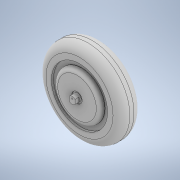
# Autodesk Inventor part: motor at24v
Saved by Autodesk Inventor 2022.2 (Build 262287010, 287A)
## iProperties
Created: 2022-03-16
Part Number: motor at24v
Material: Generic
Document SubType Name: Modeling
Designer: Finn Oriwohl
Density: 1 g/cm^3
Appearance: Default
Author: Finn Oriwohl
Autodesk Inventor part; units mm, degrees
ref_plane "YZ Plane" through (0, 0, 0) normal (1, 0, 0) x (0, 1, 0)
ref_plane "XZ Plane" through (0, 0, 0) normal (0, 1, 0) x (-1, 0, 0)
ref_plane "XY Plane" through (0, 0, 0) normal (0, 0, 1) x (1, 0, 0)
sketch "Sketch1" plane through (0, 0, 0) normal (0, 0, 1) x (1, 0, 0)
  circle A0 centre (0, 0) radius 100
  circle A1 centre (0, 0) radius 56
  circle A2 centre (0, 0) radius 67
  circle A3 centre (0, 0) radius 7.5
  dimension "d0" = 200
  dimension "d1" = 112
  dimension "d2" = 11
  dimension "d3" = 15
  constraints: 4 centre point, 3 coincident
  measures "d0" diameter of A0
  measures "d1" diameter of A1
  measures "d2" radial gap between concentric circles of A1 A2
  measures "d3" diameter of A3
extrude "Extrusion1" [suppressed]
extrude "Extrusion2" [suppressed]
extrude "Extrusion3" [suppressed]
extrude "Extrusion4" [suppressed]
sketch "Sketch2" plane through (0, 0, 0) normal (1, 0, 0) x (0, 1, 0)
  line L0 (0, 42.5) -> (0, -42.5)
  line L1 (0, 42.5) -> (8.5, 42.5)
  line L2 (8.5, 42.5) -> (8.5, -42.5)
  line L3 (8.5, -42.5) -> (0, -42.5)
  line L4 (56, 31) -> (56, -31)
  line L5 (0, 0) -> (100, 0) construction
  line L6 (56, 31) -> (12.3593, 31)
  line L7 (56, -31) -> (12.3593, -31)
  line L8 (67, 20) -> (67, -20)
  line L9 (100, 25) -> (100, -25)
  line L10 (56, 20) -> (67, 20)
  line L11 (67, -20) -> (56, -20)
  line L12 (100, 25) -> (67, 25)
  line L13 (67, 25) -> (67, 20)
  line L14 (67, -20) -> (67, -25)
  line L15 (67, -25) -> (100, -25)
  line L16 (12.3593, 31) -> (12.3593, 29.5)
  line L17 (12.3593, 29.5) -> (8.5, 29.5)
  line L18 (12.3593, -31) -> (12.3593, -29.5)
  line L19 (12.3593, -29.5) -> (8.5, -29.5)
  point P0 (56, 0)
  point P1 (8.5, 32.5)
  point P2 (8.5, -32.5)
  point P3 (67, 0)
  point P4 (4.25, 42.5)
  dimension "d12" = 85
  dimension "d13" = 8.5
  dimension "d15" = 100
  dimension "d16" = 56
  dimension "d17" = 40
  dimension "d18" = 11
  dimension "d19" = 50
  dimension "d27" = 13
  dimension "d28" = 1.5
  constraints: 40 end point, 8 point on line, 6 perpendicular, 5 midpoint, 5 vertical, 4 horizontal, 3 symmetric about line, 2 parallel, 1 coincident
  measures "d12" distance of L0.start L0.end
  measures "d13" distance of L0.start L1.end
  measures "d15" distance of L5.end L5.start
  measures "d16" distance from line of point (0, 0) L4
  measures "d17" distance of L8.start L8.end
  measures "d18" distance between parallel lines of L4 L8
  measures "d19" distance of L9.start L9.end
  measures "d27" distance from line of point (4.25, 42.5) L17
  measures "d28" distance between parallel lines of L17 L6
revolve "Revolution1" add sketch "Sketch2" angle 360 about axis through (0, 0, 42.5) along (0, 0, -1)
fillet "Fillet1" radius 20 2 edges at (0, -100, 25) (0, -100, -25)
fillet "Fillet2" radius 10 2 edges at (0, -56, 31) (0, -56, -31)
sketch "Sketch3" plane through (0, 0, 42.5) normal (0, 0, 1) x (1, 0, 0)
  circle A0 centre (0, 0) radius 8.5
  line L0 (-6.75, 5.166) -> (-6.75, -5.166)
  line L1 (6.75, 5.166) -> (6.75, -5.166)
  circle A1 centre (0, 0) radius 8.5 projected
  circle A2 centre (0, 0) radius 8.5 projected
  line L2 (-6.75, 0) -> (6.75, 0) construction
  circle A3 centre (0, 3.5) radius 2
  circle A4 centre (0, 0) radius 8.5 projected
  point P0 (6.6019, 3.3672)
  point P1 (6.6019, -3.3672)
  point P2 (0, 5.5)
  point P3 (0, 8.5)
  dimension "d29" = 4
  dimension "d24" = 13.5
  dimension "d30" = 3
  constraints: 6 end point, 5 point on circle, 3 coincident, 3 midpoint, 1 centre point, 1 concentric, 1 parallel, 1 vertical, 1 vertical alignment, 2 other
  measures "d24" distance between parallel lines of L1 L0
  measures "d30" distance of point (0, 8.5) point (0, 5.5)
extrude "Extrusion5" cut sketch "Sketch3" against normal blind 9 contours A0 L1 | L0 A0
hole "Hole1" at (0, 3.5, 42.5) direction (0, 0, -1) diameter 3.242 depth 10 thread size "M4x0.7" class "6H" standard "ISO Metric profile"
mirror "Mirror1" about plane through (0, 0, 0) normal (0, 0, 1) of "Extrusion5", "Hole1"
body "Solid1"
